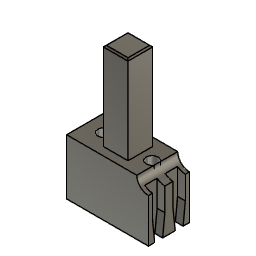
Non_movable_piece (Autodesk Fusion 360 design; units mm, degrees)
Autodesk Fusion 360 part; units mm, degrees
sketch "Sketch1" plane through (0, 0, 0) normal (0, 1, 0) x (1, 0, 0)
  line L0 (0, 0) -> (56, 0)
  line L1 (56, 0) -> (56, -38)
  line L2 (56, -38) -> (0, -38)
  line L3 (0, -38) -> (0, 0)
  line L4 (56, 0) -> (56, -1.6379)
  line L5 (56, 0) -> (56, -30)
  circle A0 centre (56, -38) radius 8
  dimension "d1" = 56
  dimension "d2" = 38
  dimension "d5" = 30
  constraint horizontal L0
  constraint vertical L1
  constraint horizontal L2
  constraint vertical L3
  constraint coincident L0.start L3.end
  constraint coincident L1 L4.end
  constraint perpendicular L0 L5
  constraint coincident L1.end L2.start
  constraint coincident L5.end A0
  measures "d1" distance of L0.start L0.end
  measures "d2" distance of L0.start L2.end
  measures "d5" distance of L0.end L5.end
  measures "d8" distance of L0.start
  measures "d9" distance of L0.start
extrude "Extrude1" add sketch "Sketch1" along normal blind 28 contours L0 L1 L2 L3 L4 L5 A0
sketch "Sketch3" plane through (0, 0, 38) normal (0, 0, 1) x (-1, 0, 0)
  line L0 (0, 0) -> (-48, 0)
  line L1 (-48, 0) -> (-48, -28)
  line L2 (-48, -28) -> (0, -28)
  line L3 (0, -28) -> (0, 0)
  line L4 (0, -28) -> (-56, -28)
  line L5 (-56, -28) -> (-56, 0)
  line L6 (-56, 0) -> (0, 0)
  line L7 (0, 0) -> (0, -28)
  line L8 (-56, -28) -> (0, 0) construction
  line L9 (0, -28) -> (-56, 0) construction
  line L10 (-36.4, -5.6) -> (-19.6, -5.6)
  line L11 (-19.6, -5.6) -> (-19.6, -22.4)
  line L12 (-19.6, -22.4) -> (-36.4, -22.4)
  line L13 (-36.4, -22.4) -> (-36.4, -5.6)
  line L14 (-36.4, -5.6) -> (-19.6, -22.4) construction
  line L15 (-19.6, -5.6) -> (-36.4, -22.4) construction
  line L16 (0, -14) -> (-56, -14) construction
  line L17 (0, -14) -> (-11.5, -14)
  line L18 (-56, -14) -> (-44.5, -14)
  circle A0 centre (-11.5, -14) radius 2
  line L19 (-28, 0) -> (-28, -28) construction
  circle A1 centre (-44.5, -14) radius 2
  circle A2 centre (-11.5, -14) radius 4.1
  circle A3 centre (-44.5, -14) radius 4.1
  line L20 (-38.15, -3.85) -> (-17.85, -3.85)
  line L21 (-17.85, -3.85) -> (-17.85, -24.15)
  line L22 (-17.85, -24.15) -> (-38.15, -24.15)
  line L23 (-38.15, -24.15) -> (-38.15, -3.85)
  line L24 (-38.15, -3.85) -> (-17.85, -24.15) construction
  line L25 (-17.85, -3.85) -> (-38.15, -24.15) construction
  line L26 (-16.35, -2.35) -> (-16.35, -25.65)
  line L27 (-16.35, -25.65) -> (-39.65, -25.65)
  line L28 (-39.65, -25.65) -> (-39.65, -2.35)
  line L29 (-39.65, -2.35) -> (-16.35, -2.35)
  point P0 (-28, -14)
  point P1 (-28, -14)
  dimension "d6" = 56
  dimension "d7" = 28
  dimension "d8" = 16.8
  dimension "d9" = 16.8
  dimension "d13" = 11.5
  dimension "d14" = 11.5
  dimension "d15" = 4
  dimension "d17" = 8.2
  dimension "d33" = 20.3
  dimension "d34" = 20.3
  dimension "d35" = -1.5
  constraint horizontal L4
  constraint vertical L5
  constraint horizontal L6
  constraint vertical L7
  constraint coincident L2.end L3.start
  constraint coincident L0.start L3.end
  constraint horizontal L10
  constraint perpendicular L10 L11
  constraint parallel L10 L12
  constraint parallel L11 L13
  constraint coincident L14 P1
  constraint coincident L15 P1
  constraint midpoint L8 P1
  constraint midpoint L7 L16.start
  constraint midpoint L5 L16.end
  constraint perpendicular L11 L17
  constraint perpendicular L1 L18
  constraint coincident L17.end A0.centre
  constraint midpoint L6 L19.start
  constraint midpoint L4 L19.end
  constraint symmetric A0 L19 A1
  constraint symmetric L19 A2 A3
  constraint horizontal L20
  constraint perpendicular L20 L21
  constraint parallel L20 L22
  constraint parallel L21 L23
  constraint coincident L24 P1
  constraint coincident L25 P1
  constraint coincident P1 P0
  measures "d6" distance of L5 L7
  measures "d7" distance of L4 L6
  measures "d8" distance of L11.end L12.end
  measures "d9" distance of L10.end L11.end
  measures "d13" distance of L16.start L17.end
  measures "d14" distance of L16.end L18.end
  measures "d15" diameter of A0
  measures "d17" diameter of A2
  measures "d33" distance of L21.end L22.end
  measures "d34" distance of L20.end L21.end
extrude "Extrude3" cut sketch "Sketch3" against normal blind 38 contours A0 | A1
extrude "Extrude2" add sketch "Sketch3" along normal blind 60 contours L10 L11 L12 L13
chamfer "Chamfer1" distance 1 angle 45 4 edges at (28, 5.6, 98) (19.6, 14, 98) (28, 22.4, 98) (36.4, 14, 98)
extrude "Extrude4" cut sketch "Sketch3" against normal blind 32 contours L1 A3 | A2
chamfer "Chamfer2" distance 1.8 angle 45 2 edges at (13.3647, 14.7232, 6) (46.3647, 14.7232, 6)
sketch "Sketch4" plane through (56, 0, 0) normal (1, 0, 0) x (0, 1, 0)
  line L0 (0, 30) -> (0, 0)
  line L1 (0, 0) -> (28, 0)
  line L2 (28, 0) -> (28, 30)
  line L3 (28, 30) -> (0, 30)
  line L4 (0, 38) -> (28, 38) construction
  line L5 (28, 38) -> (28, 0) construction
  line L6 (28, 0) -> (0, 0) construction
  line L7 (0, 0) -> (0, 38) construction
  line L8 (14, 0) -> (14, 38) construction
  line L9 (7, 0) -> (7, 38) construction
  line L10 (7, 0) -> (4.5, 0)
  line L11 (7, 14) -> (3, 14)
  line L12 (3, 14) -> (4.5, 0)
  line L13 (7, 14) -> (11, 14)
  line L14 (11, 14) -> (9.5, 0)
  line L15 (7, 0) -> (9.5, 0)
  line L16 (7, 14.2) -> (2.7774, 14.2)
  line L17 (2.7774, 14.2) -> (4.3203, -0.2)
  line L18 (7, -0.2) -> (4.3203, -0.2)
  line L19 (7, -0.2) -> (9.6797, -0.2)
  line L20 (11.2226, 14.2) -> (9.6797, -0.2)
  line L21 (7, 14.2) -> (11.2226, 14.2)
  line L22 (2.7774, 14.2) -> (2.7774, 38)
  line L23 (11.2226, 14.2) -> (11.2226, 38.0127)
  line L24 (16.7774, 14.2) -> (16.7774, 38.0127)
  line L25 (25.2226, 14.2) -> (25.2226, 38)
  line L26 (16.7774, 14.2) -> (18.3203, -0.2)
  line L27 (25.2226, 14.2) -> (23.6797, -0.2)
  line L28 (21, -0.2) -> (23.6797, -0.2)
  line L29 (21, -0.2) -> (18.3203, -0.2)
  line L30 (16.7774, 38.0127) -> (25.2226, 38)
  line L31 (11.2226, 38.0127) -> (2.7774, 38)
  dimension "d24" = 2.5
  dimension "d25" = 4
  dimension "d27" = 14
  dimension "d28" = 0.2
  dimension "d29" = 180
  dimension "d30" = 23.8127
  constraint horizontal L4
  constraint vertical L5
  constraint horizontal L6
  constraint vertical L7
  constraint coincident L1.end L2.start
  constraint midpoint L1 L8.start
  constraint midpoint L4 L8.end
  constraint perpendicular L4 L8
  constraint coincident L1 L9.start
  constraint coincident L4 L9.end
  constraint perpendicular L4 L9
  constraint perpendicular L9 L10
  constraint coincident L9 L11.start
  constraint perpendicular L9 L11
  constraint symmetric L10.start L9 L15.start
  constraint symmetric L9 L10.end L14.end
  constraint symmetric L9 L11.start L13.start
  constraint symmetric L9 L11.end L13.end
  constraint vertical L22
  constraint coincident L4 L22.end
  constraint symmetric L8 L16.end L25.start
  constraint symmetric L8 L17.end L27.end
  constraint symmetric L8 L18.start L28.start
  constraint symmetric L8 L19.end L26.end
  constraint symmetric L8 L20.start L24.start
  constraint symmetric L8 L22.end L25.end
  constraint symmetric L8 L23.end L24.end
  measures "d24" distance of L9.start L10.end
  measures "d25" distance of L11.start L11.end
  measures "d27" distance of L10 L11
  measures "d29" angle of L22 L23
  measures "d30" distance of L20.start L23.end
extrude "Extrude5" cut sketch "Sketch4" against normal blind 5.3 contours L3 L22 L23 L31 | L3 L16 L21 L22 L23 | L1 L11 L12 L13 L14 L16 L17 L20 L21 | L1 L10 L11 L12 L13 L14 L15 | L3 L24 L25 L30 | L1 L3 L24 L25 L26 L27
equation "d13 = ( 23 / 2 ) * 1 mm"
equation "d14 = ( 23 / 2 ) * 1 mm"
